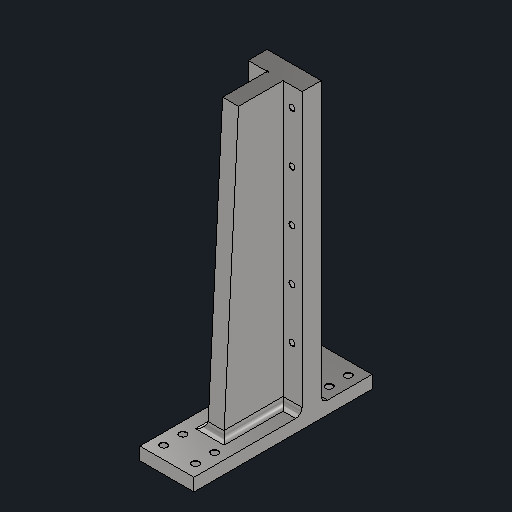
# Autodesk Inventor part: KN-00-01-04
Saved by Autodesk Inventor 2025.2 (Build 292293000, 293)
## iProperties
Created: 2025-04-28
Part Number: KN-00-01-04
Material: X5CrNi18-10
Document SubType Name: Modeling
Designer: Kacper Mik
Density: 8 g/cm^3
Appearance: Semi-Polished
Author: Kacper Mik
Autodesk Inventor part; units mm, degrees
ref_plane "YZ Plane" through (0, 0, 0) normal (1, 0, 0) x (0, 1, 0)
ref_plane "XZ Plane" through (0, 0, 0) normal (0, 1, 0) x (-1, 0, 0)
sketch "Sketch1" plane through (0, 0, 0) normal (1, 0, 0) x (0, 1, 0)
  line L0 (0, 0) -> (440, 0)
  line L1 (440, 0) -> (440, -100)
  line L2 (440, -100) -> (0, -100)
  line L3 (0, -100) -> (0, 0)
  line L4 (0, 0) -> (0, 23.0594)
  line L5 (0, 23.0594) -> (440, 0)
  dimension "d0" = 100
  dimension "d1" = 87
  dimension "d32" = 440
  constraints: 12 end point, 2 parallel, 1 horizontal, 1 perpendicular, 1 vertical
  measures "d0" distance of L0.end L1.end
  measures "d1" angle of L4 L5
  measures "d32" distance between parallel lines of L3 L1
extrude "top" add sketch "Sketch1" along normal mid plane 25
sketch "Sketch2" plane through (0, 0, 0) normal (1, 0, 0) x (0, 1, 0)
  line L0 (0, -100) -> (440, -100) projected
  line L1 (0, -100) -> (-20, -100)
  line L2 (-20, -100) -> (-20, 100)
  line L3 (-20, 100) -> (0, 100)
  line L4 (0, 100) -> (0, -100)
  point P0 (0, 0)
  dimension "d4" = 20
  dimension "d9" = 200
  constraints: 8 end point, 2 parallel, 1 horizontal, 1 perpendicular
  measures "d4" distance of L2.end L3.end
  measures "d9" distance between parallel lines of L1 L3
extrude "bott" add sketch "Sketch2" along normal mid plane 85
sketch "Sketch4" plane through (-12.5, 0, 0) normal (-1, 0, 0) x (0, 0, 1)
  line L0 (0, 440) -> (-100, 440) projected
  line L1 (-100, 0) -> (23.0594, 0) projected
  line L2 (-100, 440) -> (-70, 440)
  line L3 (-70, 440) -> (-70, 0)
  line L4 (-70, 0) -> (-100, 0)
  line L5 (-100, 0) -> (-100, 440)
  point P0 (0, 0)
  dimension "d11" = 30
  constraints: 8 end point, 2 parallel, 1 horizontal, 1 perpendicular, 1 point on line
  measures "d11" distance of L3.end L4.end
extrude "arm" add sketch "Sketch4" along normal blind 30
sketch "Sketch5" plane through (42.5, -20, -100) normal (0, 0, -1) x (-1, 0, 0)
  line L0 (0, 0) -> (0, 20) projected
  line L1 (85, 0) -> (0, 0) projected
  line L2 (0, 20) -> (85, 20)
  line L3 (85, 20) -> (85, 0)
  line L4 (85, 0) -> (0, 0)
  line L5 (0, 0) -> (0, 20)
  point P0 (42.5, 20)
  constraints: 8 end point, 2 parallel, 1 horizontal, 1 perpendicular
extrude "back" add sketch "Sketch5" along normal blind 80
sketch "Sketch8" plane through (-12.5, 440, 0) normal (0, 1, 0) x (1, 0, 0)
  line L0 (25, 0) -> (0, 0) construction
  line L1 (25, 100) -> (25, 0) construction
  line L2 (-30, 100) -> (25, 100) construction
  line L3 (-30, 70) -> (-30, 100) construction
  line L4 (0, 70) -> (-30, 70) construction
  line L5 (0, 0) -> (0, 70) construction
  line L6 (0, 71.4142) -> (-1.4142, 70)
  line L7 (-1.4142, 70) -> (0, 68.5858)
  line L8 (0, 68.5858) -> (1.4142, 70)
  line L9 (1.4142, 70) -> (0, 71.4142)
  line L10 (0, 71.4142) -> (0, 68.5858) construction
  line L11 (-1.4142, 70) -> (1.4142, 70) construction
  point P0 (12.5, 0)
  point P1 (0, 70)
  dimension "d33" = 2
  dimension "d34" = 2
  constraints: 12 end point, 2 midpoint, 2 parallel, 1 coincident, 1 perpendicular
  measures "d33" distance of L8.end L7.end
  measures "d34" distance of L7.end L6.end
ref_plane "Work Plane1" through (-276, 67.1224, -42.5) normal (0, -1, 0) x (1, 0, 0)
extrude "Extrusion7" cut sketch "Sketch8" against normal up to surface (372.8776 mm away)
sketch "Sketch9" plane through (12.5, 0, -100) normal (0, 0, -1) x (-1, 0, 0)
  circle A0 centre (331, 90) radius 5.25 construction
  circle A1 centre (331, 170) radius 5.25 construction
  circle A2 centre (331, 250) radius 5.25 construction
  circle A3 centre (331, 330) radius 5.25 construction
  circle A4 centre (331, 410) radius 5.25 construction
  circle A5 centre (39, 90) radius 5.25 construction
  circle A6 centre (39, 170) radius 5.25 construction
  circle A7 centre (39, 250) radius 5.25 construction
  circle A8 centre (39, 330) radius 5.25 construction
  circle A9 centre (39, 410) radius 5.25 construction
  circle A10 centre (147.5, 100) radius 2.567 construction
  circle A11 centre (222.5, 100) radius 2.567 construction
  circle A12 centre (147.5, 200) radius 2.567 construction
  circle A13 centre (222.5, 200) radius 2.567 construction
  circle A14 centre (147.5, 300) radius 2.567 construction
  circle A15 centre (222.5, 300) radius 2.567 construction
  circle A16 centre (147.5, 400) radius 2.567 construction
  circle A17 centre (222.5, 400) radius 2.567 construction
  line L0 (25, 60) -> (25, 440) construction
  line L1 (345, 60) -> (25, 60) construction
  line L2 (345, 440) -> (345, 60) construction
  line L3 (25, 440) -> (345, 440) construction
  constraints: 5 coincident
hole "Hole2" at (-26.5, 410, -100) at (-26.5, 330, -100) at (-26.5, 250, -100) at (-26.5, 170, -100) at (-26.5, 90, -100) direction (0, 0, 1) diameter 8.376 depth 30 thread size "M10x1.5" class "6H" standard "ISO Metric profile"
chamfer "Chamfer4" distance 0.5 angle 45 5 edges at (-26.5, 325.812, -70) (-26.5, 405.812, -70) (-26.5, 85.812, -70) (-26.5, 165.812, -70) (-26.5, 245.812, -70)
mirror "Mirror1" about plane through (0, 0, 0) normal (1, 0, 0) of "arm", "Hole2", "Chamfer4"
fillet "Fillet1" radius 10 6 edges at (27.5, 0, -70) (12.5, 0, -23.4703) (0, 0, 23.0594) (-12.5, 0, -23.4703) (-27.5, 0, -70) (0, 0, -100)
sketch "Sketch10" plane through (-42.5, 0, 100) normal (0, 1, 0) x (1, 0, 0)
  line L0 (42.5, 336) -> (42.5, -56) projected
  line L1 (85, 0) -> (0, 0) projected
  line L2 (0, 280) -> (85, 280) projected
  point P0 (42.5, 100)
  point P1 (17.5, 20)
  point P2 (67.5, 20)
  point P3 (67.5, 50)
  point P4 (17.5, 50)
  point P5 (67.5, 260)
  point P6 (17.5, 260)
  point P7 (67.5, 230)
  point P8 (17.5, 230)
  dimension "d51" = 50
  dimension "d52" = 20
  dimension "d53" = 30
  dimension "d54" = 20
  dimension "d55" = 30
  constraints: 6 vertical alignment, 4 horizontal alignment, 1 symmetric about line
  measures "d51" distance of point (67.5, 20) point (17.5, 20)
  measures "d52" distance from line of point (67.5, 20) L1
  measures "d53" distance of point (67.5, 50) point (67.5, 20)
  measures "d54" distance from line of L2 point (67.5, 260)
  measures "d55" distance of point (67.5, 230) point (67.5, 260)
hole "Hole3" at (-25, 0, 80) at (25, 0, 80) at (25, 0, 50) at (-25, 0, 50) at (25, 0, -160) at (-25, 0, -160) at (25, 0, -130) at (-25, 0, -130) direction (0, -1, 0) diameter 10.5 end through all clearance for "Socket Head Cap Screw ISO 4762" size "M10" standard "ISO"
chamfer "Chamfer5" distance 0.5 angle 45 4 edges at (-25, 0, 44.75) (25, 0, 44.75) (-25, 0, 74.75) (25, 0, 74.75)
equation "\"d55\" = d53"
body "Solid1"
